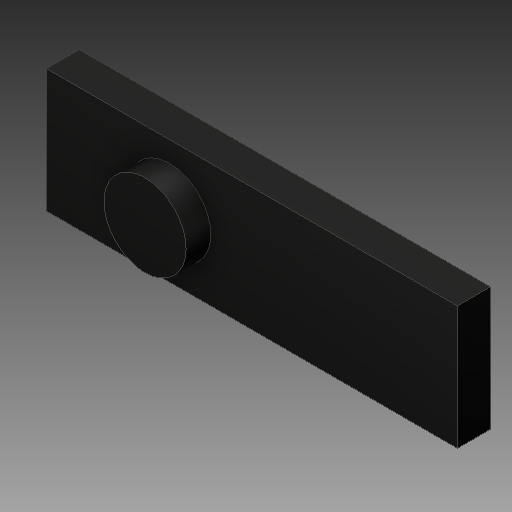
# Autodesk Inventor part: 回路.整流器
Saved by Autodesk Inventor 2019 (Build 230136000, 136)
## iProperties
Part Number: 回路.整流器
Material: 一般
Document SubType Name: Modeling
Designer: 雪村
Density: 3.0906 g/cm^3
Appearance: 光沢 - 黒
Mass: 10 g
Surface Area: 21.1425 cm^2
Volume: 3.23562 cm^3
Author: 雪村
Autodesk Inventor part; units mm, degrees
ref_plane "YZ Plane" through (0, 0, 0) normal (1, 0, 0) x (0, 1, 0)
ref_plane "XZ Plane" through (0, 0, 0) normal (0, 1, 0) x (-1, 0, 0)
ref_plane "XY Plane" through (0, 0, 0) normal (0, 0, 1) x (1, 0, 0)
sketch "スケッチ1" plane through (0, 0, 0) normal (0, 0, 1) x (1, 0, 0)
  line L0 (0, 0) -> (50, 0)
  line L1 (50, 0) -> (50, 15)
  line L2 (50, 15) -> (0, 15)
  line L3 (0, 15) -> (0, 0)
  dimension "d0" = 50
  dimension "d1" = 15
  constraints: 8 end point, 2 horizontal, 2 vertical
  measures "d0" distance of L1.end L2.end
  measures "d1" distance of L2.end L0.start
extrude "押し出し1" add sketch "スケッチ1" along normal blind 4
sketch "スケッチ2" plane through (0, 0, 4) normal (0, 0, 1) x (1, 0, 0)
  circle A0 centre (15, 7.5) radius 5
  line L0 (0, 0) -> (50, 0) projected
  line L1 (50, 0) -> (50, 15) projected
  line L2 (50, 15) -> (0, 15) projected
  line L3 (0, 15) -> (0, 0) projected
  dimension "d4" = 10
  dimension "d5" = 7.5
  dimension "d6" = 15
  constraints: 1 centre point
  measures "d4" diameter of A0
  measures "d5" distance from line of L2 A0.centre
  measures "d6" distance from line of L3 A0.centre
extrude "押し出し2" add sketch "スケッチ2" along normal blind 3 contours A0
